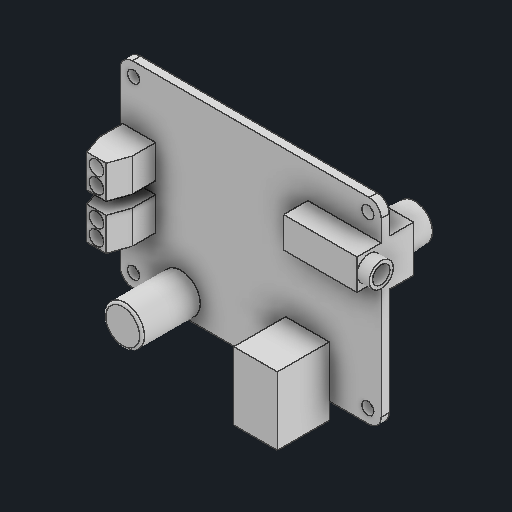
# Autodesk Inventor part: FaceAudioBoard
Saved by Autodesk Inventor 2025.2 (Build 292293000, 293)
## iProperties
Created: 2024-12-22
Part Number: FaceAudioBoard
Material: Generic
Document SubType Name: Modeling
Designer: valer
Density: 1 g/cm^3
Appearance: Default
Author: valer
Autodesk Inventor part; units mm, degrees
ref_plane "YZ Plane" through (0, 0, 0) normal (1, 0, 0) x (0, 1, 0)
ref_plane "XZ Plane" through (0, 0, 0) normal (0, 1, 0) x (-1, 0, 0)
sketch "Base" plane through (0, 0, 0) normal (0, 0, 1) x (1, 0, 0)
  line L0 (-26.9, -20.25) -> (26.9, -20.25)
  line L1 (26.9, -20.25) -> (26.9, 20.25)
  line L2 (26.9, 20.25) -> (-26.9, 20.25)
  line L3 (-26.9, 20.25) -> (-26.9, -20.25)
  line L4 (-26.9, -20.25) -> (26.9, 20.25) construction
  line L5 (26.9, -20.25) -> (-26.9, 20.25) construction
  line L6 (-25.4, 16.25) -> (-22.9, 16.25) construction
  line L7 (-22.9, 16.25) -> (-22.9, 18.75) construction
  line L8 (-22.9, 18.75) -> (-25.4, 18.75) construction
  line L9 (-25.4, 18.75) -> (-25.4, 16.25) construction
  line L10 (-25.4, 16.25) -> (-22.9, 18.75) construction
  line L11 (-22.9, 16.25) -> (-25.4, 18.75) construction
  circle A0 centre (-24.15, 17.5) radius 1.25
  line L12 (-26.9, 0) -> (0, 0) construction
  line L13 (0, 20.25) -> (0, 0) construction
  circle A1 centre (-24.15, -17.5) radius 1.25
  circle A2 centre (24.15, 17.5) radius 1.25
  circle A3 centre (24.15, -17.5) radius 1.25
  point P0 (-25.4, 17.5)
  dimension "d0" = 53.8
  dimension "d1" = 40.5
  dimension "d2" = 1.5
  dimension "d3" = 1.5
  dimension "d4" = 2.5
  constraints: 28 end point, 7 midpoint, 4 parallel, 3 centre point, 3 horizontal, 3 perpendicular, 3 symmetric about line, 1 coincident, 1 horizontal alignment, 1 vertical, 5 other
  measures "d0" distance of L1.end L2.end
  measures "d1" distance of L2.end L0.start
  measures "d2" distance between parallel lines of L2 L8
  measures "d3" distance from line of L3 point (-25.4, 17.5)
  measures "d4" distance of L6.end L7.end
extrude "BaseFeature" add sketch "Base" along normal blind 1.67
fillet "Fillet1" radius 2.5 4 edges at (-26.9, -20.25, 0.835) (26.9, -20.25, 0.835) (-26.9, 20.25, 0.835) (26.9, 20.25, 0.835)
sketch "Sketch2" plane through (0, 0, 1.67) normal (0, 0, 1) x (1, 0, 0)
  line L0 (-26.9, 17.75) -> (-26.9, -17.75) projected
  line L1 (-26.9, 0) -> (0, 0) construction
  line L2 (-26.4, 8.05) -> (-19.6, 8.05)
  line L3 (-19.6, 8.05) -> (-19.6, 1.25)
  line L4 (-19.6, 1.25) -> (-26.4, 1.25)
  line L5 (-26.4, 1.25) -> (-26.4, 8.05)
  line L6 (-26.4, -8.05) -> (-19.6, -8.05)
  line L7 (-19.6, -8.05) -> (-19.6, -1.25)
  line L8 (-19.6, -1.25) -> (-26.4, -1.25)
  line L9 (-26.4, -1.25) -> (-26.4, -8.05)
  dimension "d8" = 1.25
  dimension "d9" = 0.5
  dimension "d10" = 6.8
  constraints: 18 end point, 4 symmetric about line, 2 horizontal, 2 parallel, 2 perpendicular, 1 midpoint
  measures "d8" distance between parallel lines of L1 L4
  measures "d9" distance between parallel lines of L0 L5
  measures "d10" distance of L2.start L2.end
extrude "Extrusion2" add sketch "Sketch2" along normal blind 4.8
ref_plane "Work Plane1" through (0, 0, 10.47) normal (0, 0, 1) x (1, 0, 0)
sketch "Sketch3" plane through (0, 0, 10.47) normal (0, 0, 1) x (1, 0, 0)
  line L0 (-26.4, 8.05) -> (-19.6, 8.05) projected
  line L1 (-23, 8.05) -> (-23, 1.25) construction
  line L2 (-19.6, 1.25) -> (-26.4, 1.25) projected
  line L3 (-37.66, 0) -> (37.66, 0) construction
  line L4 (-26.4, 1.25) -> (-19.6, 1.25) projected
  line L5 (-19.6, 1.25) -> (-19.6, 8.05) projected
  line L6 (-19.6, 8.05) -> (-26.4, 8.05) projected
  line L7 (-26.4, 8.05) -> (-26.4, 1.25) projected
  line L8 (-25, 8.05) -> (-21, 8.05)
  line L9 (-21, 8.05) -> (-21, 1.25)
  line L10 (-21, 1.25) -> (-25, 1.25)
  line L11 (-25, 1.25) -> (-25, 8.05)
  point P0 (0, 0)
  dimension "d14" = 4
  constraints: 10 end point, 3 midpoint, 2 parallel, 2 point on line, 1 collinear, 1 horizontal, 1 perpendicular
  measures "d14" distance between parallel lines of L9 L11
sketch "Sketch4" plane through (0, 0, 6.47) normal (0, 0, 1) x (1, 0, 0)
  line L0 (-26.4, 1.25) -> (-19.6, 1.25) projected
  line L1 (-19.6, 1.25) -> (-19.6, 8.05) projected
  line L2 (-19.6, 8.05) -> (-26.4, 8.05) projected
  line L3 (-26.4, 8.05) -> (-26.4, 1.25) projected
  point P0 (0, 0)
loft "Loft1" add profiles "Sketch3" section 2 edges at (-23, 1.25, 6.47) (-19.6, 4.65, 6.47) (-23, 8.05, 6.47) (-26.4, 4.65, 6.47) contours L0 L9 L2 L11
mirror "Mirror1" about plane through (0, 0, 0) normal (0, 1, 0) of "Loft1"
sketch "Sketch5" plane through (-25, 1.25, 10.47) normal (0, 0, 1) x (1, 0, 0)
  line L0 (0, 6.8) -> (0, 0) projected
  line L1 (0, 0) -> (4, 0) projected
  line L2 (4, 0) -> (4, 6.8) projected
  line L3 (4, 6.8) -> (0, 6.8) projected
  line L4 (-12.66, -1.25) -> (62.66, -1.25) construction
  line L5 (2, 6.8) -> (2, 0) construction
  circle A0 centre (2, 5.025) radius 1.5
  line L6 (0, 3.4) -> (4, 3.4) construction
  circle A1 centre (2, 1.775) radius 1.5
  point P0 (25, -1.25)
  dimension "d19" = 3
  dimension "d20" = 3.25
  constraints: 4 end point, 4 midpoint, 2 centre point, 1 point on line, 1 symmetric about line, 1 other
  measures "d19" diameter of A0
  measures "d20" distance of A1.centre A0.centre
extrude "Extrusion3" cut sketch "Sketch5" against normal blind 3 contours A0 | A1
mirror "Mirror2" about plane through (0, 0, 0) normal (0, 1, 0) of "Extrusion3"
sketch "Sketch6" plane through (0, 0, 1.67) normal (0, 0, 1) x (1, 0, 0)
  line L0 (-24.4, -20.25) -> (24.4, -20.25) projected
  line L1 (-26.9, 17.75) -> (-26.9, -17.75) projected
  circle A0 centre (-14.4, -16.15) radius 4
  line L2 (-18.4, -16.15) -> (-18.4, -20.25) construction
  point P0 (0, 0)
  dimension "d23" = 8
  dimension "d24" = 4.1
  dimension "d25" = 8.5
  constraints: 2 end point, 1 horizontal alignment, 1 perpendicular, 1 point on line, 1 vertical, 2 other
  measures "d24" distance from line of L0 point (-14.4, -16.15)
  measures "d25" distance between parallel lines of L1 L2
extrude "Extrusion4" add sketch "Sketch6" along normal blind 12
fillet "Fillet2" radius 0.5 1 edges at (-18.4, -16.15, 13.67)
sketch "Sketch7" plane through (0, 0, 1.67) normal (0, 0, 1) x (1, 0, 0)
  line L0 (7.2, -9.65) -> (16.2, -9.65)
  line L1 (16.2, -9.65) -> (16.2, -23.65)
  line L2 (16.2, -23.65) -> (7.2, -23.65)
  line L3 (7.2, -23.65) -> (7.2, -9.65)
  line L4 (7.2, -23.65) -> (16.2, -23.65)
  line L5 (16.2, -23.65) -> (16.2, -20.25)
  line L6 (16.2, -20.25) -> (7.2, -20.25)
  line L7 (7.2, -20.25) -> (7.2, -23.65)
  line L8 (-24.4, -20.25) -> (24.4, -20.25) projected
  line L9 (26.9, -17.75) -> (26.9, 17.75) projected
  point P0 (0, 0)
  point P1 (11.7, -23.65)
  dimension "d29" = 9
  dimension "d30" = 14
  dimension "d31" = 3.4
  dimension "d32" = 10.7
  constraints: 16 end point, 4 parallel, 2 collinear, 2 horizontal, 2 midpoint, 2 perpendicular
  measures "d29" distance of L1.end L2.end
  measures "d30" distance of L0.end L1.end
  measures "d31" distance of L6.end L4.start
  measures "d32" distance between parallel lines of L9 L1
extrude "Extrusion5" add sketch "Sketch7" along normal blind 10.7
sketch "Sketch8" plane through (7.2, -23.65, 1.67) normal (0, -1, 0) x (1, 0, 0)
  line L0 (0, 0) -> (9, 0) projected
  line L1 (9, 0) -> (9, 10.7) projected
  line L2 (0, 10.7) -> (9, 10.7) projected
  line L3 (0, 0) -> (0, 10.7) projected
  line L4 (4.5, 10.7) -> (4.5, 0) construction
  circle A0 centre (4.5, 6.2) radius 3.85
  point P0 (-7.2, -1.67)
  dimension "d35" = 7.7
  dimension "d36" = 4.5
  constraints: 2 end point, 2 midpoint, 1 centre point, 1 point on line
  measures "d35" diameter of A0
  measures "d36" distance from line of L2 A0.centre
extrude "Extrusion6" cut sketch "Sketch8" against normal blind 10.7 contours A0
sketch "Sketch9" plane through (0, 0, 1.67) normal (0, 0, 1) x (1, 0, 0)
  line L0 (11.77, 7.05) -> (29.4, 7.05)
  line L1 (29.4, 7.05) -> (29.4, 13.37)
  line L2 (29.4, 13.37) -> (11.77, 13.37)
  line L3 (11.77, 13.37) -> (11.77, 7.05)
  line L4 (24.4, 20.25) -> (-24.4, 20.25) projected
  line L5 (26.9, 13.37) -> (26.9, 7.05)
  line L6 (26.9, -17.75) -> (26.9, 17.75) projected
  point P0 (0, 0)
  dimension "d39" = 13.2
  dimension "d40" = 6.32
  dimension "d41" = 17.63
  dimension "d42" = 2.5
  constraints: 10 end point, 2 parallel, 2 point on line, 1 collinear, 1 horizontal, 1 perpendicular, 1 vertical
  measures "d39" distance between parallel lines of L4 L0
  measures "d40" distance of L2.end L0.start
  measures "d41" distance of L1.end L2.end
  measures "d42" distance between parallel lines of L1 L5
extrude "Extrusion7" add sketch "Sketch9" along normal blind 5 contours L3 L2 L5 L0
sketch "Sketch10" plane through (26.9, -17.75, 0) normal (1, 0, 0) x (0, 0, -1)
  line L0 (-1.67, 24.8) -> (-6.67, 24.8) construction
  line L1 (-1.67, 31.12) -> (-6.67, 31.12) construction
  line L2 (-6.67, 24.8) -> (-1.67, 31.12) construction
  circle A0 centre (-4.17, 27.96) radius 1.8
  point P0 (0, 17.75)
  dimension "d45" = 3.6
  constraints: 2 end point, 1 centre point, 1 midpoint
  measures "d45" diameter of A0
extrude "Extrusion8" cut sketch "Sketch10" against normal blind 5
sketch "Sketch11" plane through (26.9, -17.75, 0) normal (1, 0, 0) x (0, 0, -1)
  circle A0 centre (-4.17, 27.96) radius 1.8 projected
  line L0 (-6.67, 24.8) -> (-6.67, 31.12) projected
  circle A1 centre (-4.17, 27.96) radius 2.5
  point P0 (0, 17.75)
  constraints: 1 centre point, 1 coincident
extrude "Extrusion9" add sketch "Sketch11" along normal blind 2.5
sketch "Sketch12" plane through (0, 0, 0) normal (0, 0, -1) x (-1, 0, 0)
  line L0 (-26.9, 13.75) -> (-17.4, 13.75)
  line L1 (-17.4, 13.75) -> (-17.4, 4.25)
  line L2 (-17.4, 4.25) -> (-26.9, 4.25)
  line L3 (-26.9, 4.25) -> (-26.9, 13.75)
  line L4 (-26.9, -17.75) -> (-26.9, 17.75) projected
  line L5 (-24.4, 20.25) -> (24.4, 20.25) projected
  point P0 (0, 0)
  dimension "d50" = 9.5
  dimension "d51" = 6.5
  constraints: 8 end point, 2 parallel, 2 perpendicular, 1 collinear, 1 horizontal
  measures "d50" distance of L2.end L0.start
  measures "d51" distance between parallel lines of L5 L0
extrude "Extrusion10" add sketch "Sketch12" along normal blind 5
sketch "Sketch13" plane through (0, 0, -5) normal (0, 0, -1) x (-1, 0, 0)
  line L0 (-17.4, 13.75) -> (-26.9, 13.75) projected
  line L1 (-26.9, 13.75) -> (-26.9, 4.25) projected
  line L2 (-26.9, 4.25) -> (-17.4, 4.25) projected
  line L3 (-17.4, 4.25) -> (-17.4, 13.75) projected
  circle A0 centre (-22.15, 9) radius 4
  line L4 (-17.4, 13.75) -> (-17.4, 4.25) projected
  line L5 (-26.9, 13.75) -> (-17.4, 4.25) construction
  point P0 (0, 0)
  dimension "d54" = 8
  constraints: 2 end point, 1 centre point, 1 coincident, 1 midpoint
  measures "d54" diameter of A0
extrude "Extrusion11" add sketch "Sketch13" along normal blind 5 draft -4 contours A0
body "Solid1"
